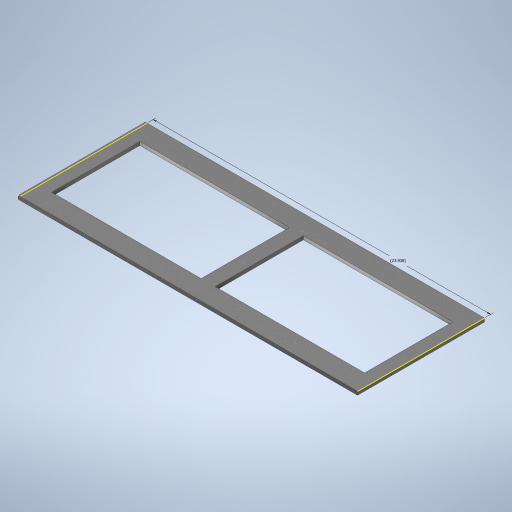
# Autodesk Inventor part: BottomHalfofFront_Ocampo
Saved by Autodesk Inventor 2023 (Build 270158000, 158)
## iProperties
Created: 2025-03-05
Part Number: BottomHalfofFront_Ocampo
Material: Generic
Document SubType Name: Modeling
Designer: FrameUser
Density: 1 g/cm^3
Appearance: Default
Author: FrameUser
Autodesk Inventor part; units mm, degrees
ref_plane "YZ Plane" through (0, 0, 0) normal (1, 0, 0) x (0, 1, 0)
ref_plane "XZ Plane" through (0, 0, 0) normal (0, 1, 0) x (-1, 0, 0)
ref_plane "XY Plane" through (0, 0, 0) normal (0, 0, 1) x (1, 0, 0)
sketch "Sketch1" plane through (0, 0, 0) normal (0, 1, 0) x (-1, 0, 0)
  line L0 (0, 0) -> (-614.3625, 0)
  line L1 (-614.3625, 0) -> (-614.3625, -228.6)
  line L2 (-614.3625, -228.6) -> (0, -228.6)
  line L3 (0, -228.6) -> (0, 0)
  dimension "d0" = 614.3625
  dimension "d1" = 228.6
  constraints: 8 end point, 2 perpendicular, 1 horizontal, 1 vertical
  measures "d0" distance of L0.start L0.end
  measures "d1" distance of L0.end L1.end
extrude "Extrusion1" add sketch "Sketch1" along normal blind 6.35
sketch "Sketch2" plane through (0, 6.35, 0) normal (0, 1, 0) x (1, 0, 0)
  line L0 (0, 228.6) -> (0, 0) projected
  line L1 (0, 0) -> (307.1812, 0)
  line L2 (0, 0) -> (614.3625, 0) projected
  line L3 (307.1812, 0) -> (307.1812, 226.2221)
  line L4 (0, 0) -> (25.4, 0)
  line L5 (25.4, 0) -> (25.4, 25.4)
  line L6 (25.4, 25.4) -> (294.4812, 25.4)
  line L7 (294.4812, 25.4) -> (294.4812, 203.2)
  line L8 (294.4812, 203.2) -> (25.4, 203.2)
  line L9 (25.4, 203.2) -> (25.4, 25.4)
  line L10 (588.9625, 25.4) -> (319.8812, 25.4)
  line L11 (319.8812, 25.4) -> (319.8812, 203.2)
  line L12 (319.8812, 203.2) -> (588.9625, 203.2)
  line L13 (588.9625, 203.2) -> (588.9625, 25.4)
  dimension "d4" = 307.1812
  dimension "d5" = 25.4
  dimension "d6" = 25.4
  dimension "d7" = 269.0813
  dimension "d8" = 177.8
  constraints: 24 end point, 5 perpendicular, 4 symmetric about line, 2 point on line, 1 midpoint, 1 parallel
  measures "d4" distance of L0.end L1.end
  measures "d5" distance of L0.end L4.end
  measures "d6" distance of L4.end L5.end
  measures "d7" distance of L5.end L6.end
  measures "d8" distance of L6.end L7.end
extrude "Extrusion2" cut sketch "Sketch2" against normal blind 117.475
sketch "Sketch3" plane through (0, 6.35, 0) normal (0, 1, 0) x (1, 0, 0)
  line L0 (614.3625, 228.6) -> (0, 228.6) projected
  line L1 (0, 228.6) -> (3.175, 228.6)
  line L2 (3.175, 228.6) -> (3.175, 0)
  line L3 (3.175, 0) -> (0, 0)
  line L4 (0, 0) -> (3.175, 0)
  line L5 (0, 228.6) -> (0, 0) projected
  line L6 (0, 228.6) -> (0, 0)
  dimension "d11" = 3.175
  constraints: 10 end point, 2 collinear, 2 perpendicular, 1 point on line
  measures "d11" distance of L0.end L1.end
sketch "Sketch4" plane through (0, 6.35, 0) normal (0, 1, 0) x (1, 0, 0)
  line L0 (614.3625, 0) -> (614.3625, 228.6) projected
  line L1 (614.3625, 228.6) -> (611.1875, 228.6)
  line L2 (614.3625, 228.6) -> (0, 228.6) projected
  line L3 (611.1875, 228.6) -> (611.1875, 0)
  line L4 (611.1875, 0) -> (614.3625, 0)
  line L5 (614.3625, 0) -> (611.1875, 0)
  line L6 (614.3625, 228.6) -> (614.3625, 0)
  line L7 (294.4812, 25.4) -> (25.4, 25.4) projected
  line L8 (25.4, 203.2) -> (294.4812, 203.2) projected
  line L9 (294.4812, 203.2) -> (294.4812, 25.4) projected
  line L10 (25.4, 25.4) -> (25.4, 203.2) projected
  line L11 (25.4, 25.4) -> (25.4, 34.925)
  line L12 (25.4, 34.925) -> (294.4812, 34.925)
  line L13 (294.4812, 25.4) -> (294.4812, 34.925)
  line L14 (294.4812, 25.4) -> (25.4, 25.4)
  line L15 (25.4, 203.2) -> (294.4812, 203.2)
  line L16 (294.4812, 203.2) -> (294.4812, 193.675)
  line L17 (294.4812, 193.675) -> (25.4, 193.675)
  line L18 (25.4, 203.2) -> (25.4, 193.675)
  point P0 (0, 0)
  dimension "d12" = 3.175
  dimension "d20" = 177.8
  dimension "d21" = 269.0813
  dimension "d22" = 9.525
  dimension "d23" = 9.525
  constraints: 26 end point, 5 collinear, 5 point on line, 4 perpendicular, 1 parallel
  measures "d12" distance of L0.end L1.end
  measures "d20" distance between parallel lines of L7 L8
  measures "d21" distance between parallel lines of L9 L10
  measures "d22" distance of L7.end L11.end
  measures "d23" distance of L8.end L16.end
sketch "Sketch5" plane through (0, 6.35, 0) normal (0, 1, 0) x (1, 0, 0)
  line L0 (614.3625, 228.6) -> (0, 228.6) projected
  line L1 (0, 0) -> (614.3625, 0) projected
  line L2 (0, 228.6) -> (3.175, 228.6)
  line L3 (3.175, 228.6) -> (3.175, 0)
  line L4 (3.175, 0) -> (0, 0)
  line L5 (0, 0) -> (0, 228.6)
  line L6 (614.3625, 228.6) -> (611.1875, 228.6)
  line L7 (611.1875, 228.6) -> (611.1875, 0)
  line L8 (611.1875, 0) -> (614.3625, 0)
  line L9 (614.3625, 0) -> (614.3625, 228.6)
  dimension "d13" = 3.175
  dimension "d14" = 3.175
  constraints: 16 end point, 4 parallel, 2 horizontal, 2 perpendicular, 2 point on line
  measures "d13" distance of L3.end L4.end
  measures "d14" distance of L8.end L7.end
extrude "Extrusion3" cut sketch "Sketch5" against normal blind 25.4 contours L3 L1 L5 L0
sketch "Sketch6" plane through (0, 6.35, 0) normal (0, 1, 0) x (1, 0, 0)
  line L0 (3.175, 0) -> (614.3625, 0) projected
  line L1 (614.3625, 228.6) -> (611.1875, 228.6)
  line L2 (611.1875, 228.6) -> (611.1875, 0)
  line L3 (611.1875, 0) -> (614.3625, 0)
  line L4 (614.3625, 0) -> (614.3625, 228.6)
  point P0 (0, 0)
  dimension "d17" = 3.175
  constraints: 8 end point, 2 parallel, 1 horizontal, 1 perpendicular, 1 point on line
  measures "d17" distance of L3.end L2.end
extrude "Extrusion4" cut sketch "Sketch6" against normal blind 25.4
extrude "Extrusion5" add sketch "Sketch4" against normal blind 6.35 contours L7 L10 L12 L9 | L17 L10 L8 L9
sketch "Sketch7" plane through (0, 6.35, 0) normal (0, 1, 0) x (1, 0, 0)
  line L0 (319.8812, 203.2) -> (319.8812, 25.4) projected
  line L1 (319.8812, 203.2) -> (319.8812, 193.675)
  line L2 (319.8812, 193.675) -> (588.9625, 193.675)
  line L3 (588.9625, 25.4) -> (588.9625, 203.2) projected
  line L4 (588.9625, 203.2) -> (588.9625, 193.675)
  line L5 (588.9625, 203.2) -> (319.8812, 203.2) projected
  line L6 (588.9625, 203.2) -> (319.8812, 203.2)
  line L7 (319.8812, 25.4) -> (588.9625, 25.4) projected
  line L8 (319.8812, 25.4) -> (319.8812, 34.925)
  line L9 (319.8812, 34.925) -> (588.9625, 34.925)
  line L10 (588.9625, 25.4) -> (588.9625, 34.925)
  line L11 (588.9625, 25.4) -> (319.8812, 25.4)
  point P0 (0, 0)
  dimension "d26" = 9.525
  dimension "d27" = 9.525
  constraints: 16 end point, 4 point on line, 3 perpendicular, 2 parallel, 1 collinear
  measures "d26" distance of L0.start L1.end
  measures "d27" distance of L0.end L8.end
extrude "Extrusion6" add sketch "Sketch7" against normal blind 6.35 contours L5 L3 L2 L0 | L9 L3 L7 L0
sketch "Sketch8" plane through (0, 6.35, 0) normal (0, 1, 0) x (1, 0, 0)
  line L0 (611.1875, 0) -> (611.1875, 228.6) projected
  line L1 (3.175, 228.6) -> (3.175, 0) projected
  point P0 (0, 0)
  dimension "d30" = 608.0125
  measures "d30" distance between parallel lines of L0 L1
extrude "Extrusion7" add sketch "Sketch3" against normal blind 6.35
body "Solid1"
